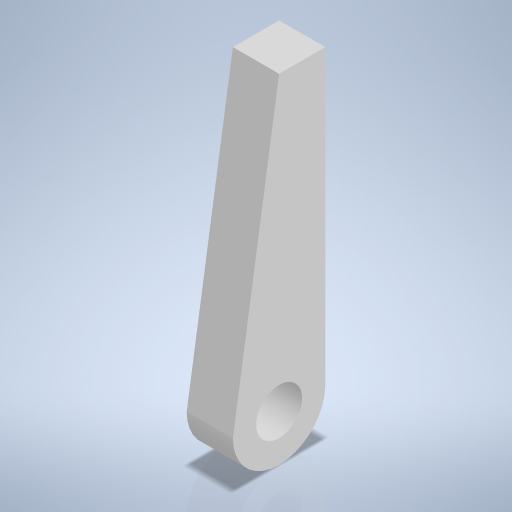
# Autodesk Inventor part: 109 part 2
Saved by Autodesk Inventor 2024 (Build 280153000, 153)
## iProperties
Created: 2024-07-24
Part Number: 109 part 2
Material: Generisch
Document SubType Name: Modeling
Designer: ffogue
Density: 1 g/cm^3
Appearance: Vorgabe
Author: ffogue
Autodesk Inventor part; units mm, degrees
ref_plane "YZ Plane" through (0, 0, 0) normal (1, 0, 0) x (0, 1, 0)
ref_plane "XZ Plane" through (0, 0, 0) normal (0, 1, 0) x (-1, 0, 0)
ref_plane "XY Plane" through (0, 0, 0) normal (0, 0, 1) x (1, 0, 0)
sketch "Skizze1" plane through (0, 0, 0) normal (1, 0, 0) x (0, 1, 0)
  line L0 (0, 0) -> (3, 0)
  line L1 (3, 0) -> (3, -19)
  arc A0 (-3, -19) -> (3, -19) centre (0, -19) ccw
  line L2 (-3, -19) -> (0, 0)
  dimension "d0" = 3
  dimension "d1" = 19
  dimension "d2" = 3
  dimension "d3" = 3
  constraints: 6 end point, 2 point on circle, 1 centre point, 1 horizontal, 1 horizontal alignment, 1 perpendicular, 1 tangent, 1 vertical alignment
  measures "d0" radius of A0
  measures "d1" distance from line of A0.centre L0
  measures "d2" distance from line of L1 A0.centre
  measures "d3" distance of L0.start L0.end
extrude "Extrusion1" add sketch "Skizze1" along normal blind 3
sketch "Skizze2" plane through (3, 0, 0) normal (1, 0, 0) x (0, 0, -1)
  arc A0 (19, -3) -> (19, 3) centre (19, 0) ccw projected
  point P0 (0, 0)
  constraints: 1 coincident
hole "Bohrung1" at (3, 0, -19) direction (-1, 0, 0) diameter 3 depth 3
